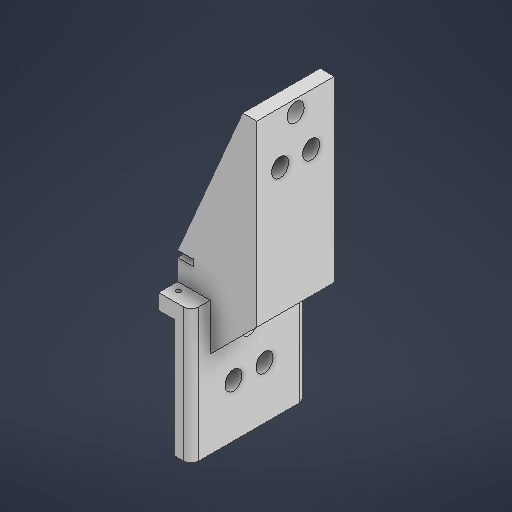
# Autodesk Inventor part: Camera Bracket
Saved by Autodesk Inventor 2025 (Build 290162000, 162)
## iProperties
Created: 2025-02-14
Part Number: Camera Bracket
Material: Generic
Document SubType Name: Modeling
Designer: mayhe
Density: 1 g/cm^3
Appearance: Default
Author: mayhe
Autodesk Inventor part; units mm, degrees
note: some values were not read from the file. Chosen so that the rebuilt part matches the saved one: edges of "Chamfer2".
sketch "Sketch1" plane through (0, 0, 0) normal (0, 1, 0) x (-1, 0, 0)
  line L0 (5.5, 37.25) -> (-5.5, 37.25)
  line L1 (-5.5, 37.25) -> (-5.5, -37.25)
  line L2 (-5.5, -37.25) -> (5.5, -37.25)
  line L3 (5.5, -37.25) -> (5.5, 37.25)
  line L4 (5.5, 37.25) -> (-5.5, -37.25) construction
  line L5 (-5.5, 37.25) -> (5.5, -37.25) construction
  circle A0 centre (0, 30) radius 1.5
  line L6 (5.5, 0) -> (-5.5, 0)
  circle A1 centre (0, -30) radius 1.5
  line L7 (-5.5, -25) -> (5.5, -25)
  line L8 (5.5, -25) -> (5.5, 25)
  line L9 (5.5, 25) -> (-5.5, 25)
  line L10 (-5.5, 25) -> (-5.5, -25)
  line L11 (-5.5, -25) -> (5.5, 25) construction
  line L12 (5.5, -25) -> (-5.5, 25) construction
  point P0 (0, 0)
  dimension "d0" = 11
  dimension "d1" = 74.5
  dimension "d2" = 3
  dimension "d3" = 7.25
  dimension "d28" = 50
  constraints: 26 end point, 6 midpoint, 4 parallel, 2 centre point, 2 horizontal, 2 perpendicular, 1 point on line, 1 symmetric about line, 1 other
  measures "d0" distance of L2.end L1.end
  measures "d1" distance of L1.end L0.end
  measures "d2" diameter of A0
  measures "d3" distance from line of L0 A0.centre
  measures "d28" distance of L8.end L7.end
extrude "Extrusion1" add sketch "Sketch1" along normal blind 10
sketch "Sketch2" plane through (5.5, 0, 37.25) normal (1, 0, 0) x (0, 0, -1)
  line L0 (0, 10) -> (74.5, 10) projected
  line L1 (0, 0) -> (74.5, 0) projected
  line L2 (0, 10) -> (74.5, 10)
  line L3 (74.5, 10) -> (74.5, 0)
  line L4 (74.5, 0) -> (0, 0)
  line L5 (0, 0) -> (0, 10)
  point P0 (37.25, 0)
  constraints: 8 end point, 2 parallel, 1 horizontal, 1 perpendicular
extrude "Extrusion2" add sketch "Sketch2" along normal blind 10
sketch "Sketch3" plane through (0, 0, 0) normal (0, -1, 0) x (1, 0, 0)
  line L0 (-5.5, 37.25) -> (15.5, 37.25) projected
  line L1 (-5.5, -37.25) -> (15.5, -37.25) projected
  line L2 (15.5, 37.25) -> (4.8, 37.25)
  line L3 (4.8, 37.25) -> (4.8, -37.25)
  line L4 (4.8, -37.25) -> (15.5, -37.25)
  line L5 (15.5, -37.25) -> (15.5, 37.25)
  point P0 (0, 0)
  dimension "d9" = 10.7
  constraints: 8 end point, 2 parallel, 1 horizontal, 1 perpendicular, 1 point on line
  measures "d9" distance of L4.end L3.end
extrude "Extrusion3" add sketch "Sketch3" along normal blind 76
ref_plane "Work Plane1" through (15.5, -76, -37.25) normal (-0.9081432, 0.4186597, 0) x (0, 0, 1)
ref_plane "Work Plane3" through (10.9593, -73.9067, -37.25) normal (-0.9081432, 0.4186597, 0) x (0, 0, 1)
sketch "Sketch4" plane through (10.9593, -73.9067, -37.25) normal (-0.9081432, 0.4186597, 0) x (0, 0, 1)
  circle A0 centre (37.25, 54.5) radius 2
  circle A1 centre (37.25, 54.5) radius 5.5
  circle A2 centre (27.25, 30.8) radius 2
  circle A3 centre (27.25, 30.8) radius 5.5
  line L0 (37.25, 62.5297) -> (37.25, 0)
  line L1 (0, 0) -> (74.5, 0) projected
  circle A4 centre (47.25, 30.8) radius 5.5
  circle A5 centre (47.25, 30.8) radius 2
  point P0 (37.25, 0)
  dimension "d13" = 4
  dimension "d14" = 11
  dimension "d15" = 4
  dimension "d16" = 11
  dimension "d19" = 10
  dimension "d20" = 23.7
  dimension "d23" = 54.5
  constraints: 6 centre point, 3 coincident, 2 end point, 2 midpoint, 2 symmetric about line, 2 other
  measures "d13" diameter of A0
  measures "d14" diameter of A1
  measures "d15" diameter of A2
  measures "d16" diameter of A3
  measures "d19" horizontal distance of A3.centre A0.centre
  measures "d20" vertical distance of A3.centre A0.centre
  measures "d23" distance of point (37.25, 0) A0.centre
extrude "Extrusion4" cut sketch "Sketch4" along normal blind 15 contours A0 L0 | A0 L0 A1 | L0 A0 | A0 L0 A1 | A2 | A3 | A4 | A5
extrude "Extrusion11" cut sketch "Sketch4" along normal blind 25.925 contours A0 L0 | A0 L0 A1 | L0 A0 | A0 L0 A1
extrude "Extrusion6" cut sketch "Sketch4" along normal through all contours A0 L0 | L0 A0 | A2 | A5
extrude "Extrusion7" add sketch "Sketch1" along normal blind 125 contours L3 L6 L1 L9 | L3 L7 L1 L6
sketch "Sketch5" plane through (5.5, 10, -25) normal (1, 0, 0) x (0, 0, -1)
  line L0 (0, 115) -> (-50, 115) projected
  line L1 (0, 0) -> (0, 115) projected
  line L2 (-50, 115) -> (0, 115)
  line L3 (0, 115) -> (0, 0)
  line L4 (0, 0) -> (-50, 0)
  line L5 (-50, 0) -> (-50, 115)
  point P0 (-25, -10)
  constraints: 8 end point, 2 parallel, 1 horizontal, 1 perpendicular
extrude "Extrusion8" add sketch "Sketch5" along normal blind 40
chamfer "Chamfer1" distance 40 angle 23.25 1 edges at (-5.5, 125, 0) measured on face at (-5.5, 48.3333, -8.3333)
sketch "Sketch6" plane through (11.6854, 125, -25) normal (-0.9187912, 0.3947439, 0) x (0, 0, 1)
  circle A0 centre (25, 6.4645) radius 2
  circle A1 centre (25, 6.4645) radius 5.5
  circle A2 centre (15, -17.2355) radius 5.5
  circle A3 centre (15, -17.2355) radius 2
  line L0 (25, 14.6915) -> (25, -47.8381)
  circle A4 centre (35, -17.2355) radius 5.5
  circle A5 centre (35, -17.2355) radius 2
  line L1 (0, -43.5355) -> (50, -43.5355) projected
  point P0 (25, -119.4616)
  point P1 (25, -43.5355)
  point P2 (25, -43.5355)
  dimension "d36" = 4
  dimension "d37" = 11
  dimension "d38" = 4
  dimension "d39" = 11
  dimension "d40" = 10
  dimension "d41" = 23.7
  dimension "d44" = 50
  constraints: 6 centre point, 3 coincident, 2 end point, 2 midpoint, 2 symmetric about line, 2 vertical alignment, 1 vertical, 2 other
  measures "d36" diameter of A0
  measures "d37" diameter of A1
  measures "d38" diameter of A3
  measures "d39" diameter of A2
  measures "d40" horizontal distance of A2.centre A0.centre
  measures "d41" vertical distance of A2.centre A0.centre
  measures "d44" distance from line of L1 A0.centre
extrude "Extrusion9" cut sketch "Sketch6" against normal through all contours A0 L0 | L0 A0 | A3 | A5
chamfer "Chamfer2" distance 30 distance2 30 1 edges at (15.5, 10, 0)
sketch "Sketch8" plane through (11.6854, 125, -25) normal (-0.9187912, 0.3947439, 0) x (0, 0, 1)
  line L0 (0, 0) -> (0, 13.3481) projected
  line L1 (-12.25, -121.6327) -> (62.25, -121.6327) projected
  line L2 (0, 13.3481) -> (50, 13.3481)
  line L3 (50, 13.3481) -> (50, -121.6327)
  line L4 (50, -121.6327) -> (0, -121.6327)
  line L5 (0, -121.6327) -> (0, 13.3481)
  point P0 (25, -119.4616)
  point P1 (0, 0)
  dimension "d59" = 50
  constraints: 8 end point, 2 parallel, 1 horizontal, 1 perpendicular, 1 point on line
  measures "d59" distance of L3.end L4.end
extrude "Extrusion12" cut sketch "Sketch8" against normal blind 22.7
ref_plane "Work Plane4" through (64.6996, 102.2233, -25) normal (-0.9187912, 0.3947439, 0) x (0, 0, 1)
sketch "Sketch9" plane through (64.6996, 102.2233, -25) normal (-0.9187912, 0.3947439, 0) x (0, 0, 1)
  circle A0 centre (35, -17.2355) radius 2 projected
  circle A1 centre (35, -17.2355) radius 5.5
  circle A2 centre (15, -17.2355) radius 2 projected
  circle A3 centre (15, -17.2355) radius 5.5
  circle A4 centre (25, 6.4645) radius 2 projected
  circle A5 centre (25, 6.4645) radius 5.5
  point P0 (25, -119.4616)
  dimension "d63" = 11
  dimension "d64" = 11
  dimension "d65" = 11
  constraints: 3 centre point, 3 coincident
  measures "d63" diameter of A1
  measures "d64" diameter of A3
  measures "d65" diameter of A5
extrude "Extrusion13" cut sketch "Sketch9" along normal blind 28.9375 contours A0 | A1 | A2 | A3 | A4 | A5
ref_plane "Work Plane5" through (32.5419, 116.0393, -25) normal (-0.9187912, 0.3947439, 0) x (0, 0, 1)
ref_plane "Work Plane6" through (-5.5, 27.4944, -18.625) normal (0.3947439, 0.9187912, 0) x (0, 0, -1)
sketch "Sketch10" plane through (-5.5, 27.4944, -18.625) normal (0.3947439, 0.9187912, 0) x (0, 0, -1)
  circle A0 centre (-18.625, 15) radius 25
  line L0 (-43.625, 0) -> (6.375, 0) projected
  point P0 (-18.625, -15.9066)
  point P1 (-38.625, 0)
  point P2 (1.375, 0)
  dimension "d70" = 50
  dimension "d71" = 15
  constraints: 1 centre point
  measures "d70" diameter of A0
  measures "d71" distance from line of L0 A0.centre
extrude "Extrusion14" cut sketch "Sketch10" along normal blind 70.5 and the other way blind 54.3375
sketch "Sketch11" plane through (15.5, 10, -25) normal (0, 0, -1) x (-1, 0, 0)
  line L0 (21, 17.4944) -> (-6.8294, 82.2691) projected
  line L1 (21, 17.4944) -> (11, 17.4944)
  line L2 (11, 17.4944) -> (11, 13.4944)
  line L3 (11, 13.4944) -> (21, 13.4944)
  line L4 (21, 13.4944) -> (21, 17.4944)
  point P0 (15.5, -10)
  dimension "d76" = 10
  dimension "d77" = 4
  constraints: 8 end point, 2 parallel, 1 horizontal, 1 perpendicular
  measures "d76" distance of L3.end L2.end
  measures "d77" distance of L2.end L1.end
extrude "Extrusion15" cut sketch "Sketch11" against normal blind 70.5
fillet "Fillet1" radius 5 2 edges at (15.5, -33, 37.25) (15.5, -33, -37.25)
body "Solid1"
